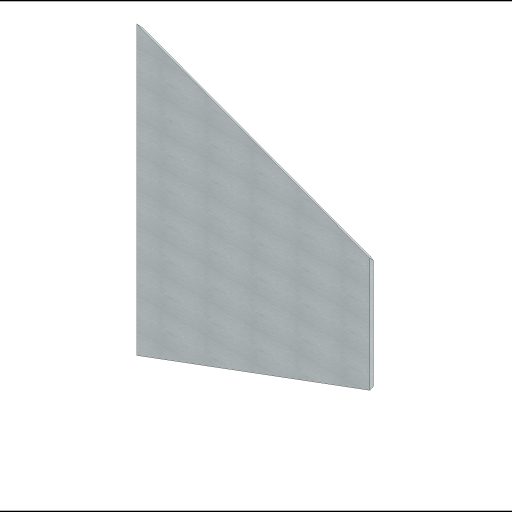
# Autodesk Inventor part: Wind Tunnel Inlet Body Single Panel
Saved by Autodesk Inventor 2023 (Build 270158000, 158)
## iProperties
Created: 2022-01-10
Part Number: Wind Tunnel Inlet Body Single Panel
Material: Wood (Oak)
Document SubType Name: Modeling
Designer: kamer
Density: 0.76 g/cm^3
Appearance: Wood - Painted White
Author: kamer
Autodesk Inventor part; units mm, degrees
ref_plane "YZ Plane" through (0, 0, 0) normal (1, 0, 0) x (0, 1, 0)
sketch "Sketch1" plane through (0, 0, 0) normal (0, 0, 1) x (1, 0, 0)
  line L0 (0, 0) -> (685.8, 0)
  line L1 (685.8, 0) -> (685.8, 838.2)
  line L2 (685.8, 838.2) -> (0, 838.2)
  line L3 (0, 838.2) -> (0, 0)
  line L4 (685.8, 254) -> (787.4, 254) construction
  line L5 (787.4, 254) -> (787.4, 584.2) construction
  line L6 (787.4, 584.2) -> (685.8, 584.2) construction
  line L7 (0, 838.2) -> (685.8, 584.2)
  line L8 (0, 0) -> (685.8, 254)
  dimension "d0" = 685.8
  dimension "d1" = 838.2
  dimension "d2" = 101.6
  dimension "d3" = 330.2
  dimension "d4" = 254
  constraints: 18 end point, 4 perpendicular, 2 parallel, 2 point on line, 1 horizontal
  measures "d0" distance of L2.end L1.end
  measures "d1" distance of L1.end L0.end
  measures "d2" distance of L4.start L4.end
  measures "d3" distance of L4.end L5.end
  measures "d4" distance between parallel lines of L0 L4
extrude "Extrusion1" add sketch "Sketch1" along normal blind 12.7 contours L3 L7 L1 L8
sketch "Sketch2" plane through (0, 0, 0) normal (-1, 0, 0) x (0, 0, 1)
  line L0 (12.7, 838.2) -> (12.7, 0) projected
  line L1 (12.7, 0) -> (0, 11.7954)
  line L2 (0, 838.2) -> (0, 0) projected
  line L3 (12.7, 0) -> (30.0327, 0) construction
  line L4 (12.7, 838.2) -> (0, 825.5)
  line L5 (12.7, 838.2) -> (30.6605, 838.2) construction
  line L6 (0, 838.2) -> (12.7, 838.2) projected
  line L7 (12.7, 838.2) -> (0, 838.2)
  line L8 (0, 838.2) -> (0, 825.5)
  line L9 (0, 0) -> (12.7, 0) projected
  line L10 (12.7, 0) -> (0, 0)
  line L11 (0, 0) -> (0, 11.7954)
  dimension "d7" = 137.115
  dimension "d8" = 135
  constraints: 16 end point, 3 horizontal, 2 equal length, 2 perpendicular, 2 point on line, 1 collinear
  measures "d7" angle of L3 L1
  measures "d8" angle of L4 L5
sketch "Sketch3" plane through (685.8, 254, 0) normal (1, 0, 0) x (0, 0, -1)
  line L0 (-12.7, -254) -> (-12.7, 0) projected
  line L1 (-12.7, 0) -> (0, 11.7954)
  line L2 (0, 0) -> (0, 330.2) projected
  line L3 (-12.7, 0) -> (4.6327, 0) construction
  line L4 (0, 11.7954) -> (0, 0)
  line L5 (0, 0) -> (-12.7, 0)
  line L6 (-12.7, 0) -> (-12.7, 330.2) projected
  line L7 (-12.7, 330.2) -> (0, 316.526)
  line L8 (0, 316.526) -> (0, 330.2)
  line L9 (0, 330.2) -> (-12.7, 330.2)
  point P0 (0, -254)
  dimension "d9" = 42.885
  constraints: 14 end point, 3 perpendicular, 3 point on line, 1 collinear, 1 equal length, 1 horizontal
  measures "d9" angle of L3 L1
loft "Loft1" cut profiles "Sketch3", "Sketch2" contours L1 L2 L5 / L9 L2 L1
sketch "Sketch4" plane through (685.8, 584.2, 12.7) normal (1, 0, 0) x (0, 0, -1)
  line L0 (0, 0) -> (0, 254) projected
  line L1 (0, 0) -> (12.7, -11.7954)
  line L2 (12.7, -318.4046) -> (12.7, 0) projected
  line L3 (0, 0) -> (17.3327, 0) construction
  line L4 (12.7, -11.7954) -> (12.7, 0)
  line L5 (12.7, 0) -> (0, 0)
  point P0 (12.7, -584.2)
  dimension "d14" = 42.885
  constraints: 8 end point, 1 collinear, 1 equal length, 1 horizontal, 1 perpendicular, 1 point on line
  measures "d14" angle of L1 L3
sketch "Sketch5" plane through (0, 11.7954, 0) normal (-1, 0, 0) x (0, 0, 1)
  line L0 (0, 826.4046) -> (12.7, 826.4046) projected
  line L1 (12.7, 826.4046) -> (0, 814.6093)
  line L2 (0, 572.4046) -> (0, 826.4046) projected
  line L3 (12.7, 826.4046) -> (30.0327, 826.4046) construction
  line L4 (0, 814.6093) -> (0, 826.4046)
  line L5 (0, 826.4046) -> (12.7, 826.4046)
  point P0 (0, -11.7954)
  dimension "d15" = 137.115
  constraints: 8 end point, 1 collinear, 1 equal length, 1 horizontal, 1 perpendicular, 1 point on line
  measures "d15" angle of L1 L3
loft "Loft2" cut profiles "Sketch5", "Sketch4"
ref_plane "Work Plane1" through (685.8, 0, 0) normal (0.923076, 0, -0.3846176) x (0, 1, 0)
ref_plane "Work Plane2" through (0, 419.1, 0) normal (0, 1, 0) x (-1, 0, 0)
sketch "Sketch7" plane through (0, 419.1, 0) normal (0, 1, 0) x (-1, 0, 0)
  line L0 (-685.8, 0) -> (0, 0) projected
  line L1 (-685.8, 0) -> (-680.7358, 12.7)
  line L2 (0, 12.7) -> (-685.8, 12.7) projected
  line L3 (-685.8, 0) -> (-672.1275, 0) construction
  line L4 (-680.7358, 12.7) -> (-685.8, 12.7)
  line L5 (-685.8, 12.7) -> (-685.8, 0)
  dimension "d26" = 68.26
  constraints: 8 end point, 1 collinear, 1 equal length, 1 horizontal, 1 perpendicular, 1 point on line
  measures "d26" angle of L3 L1
extrude "Extrusion3" cut sketch "Sketch7" against normal through all both and the other way through all
sketch "Sketch8" plane through (0, 419.1, 0) normal (0, 1, 0) x (-1, 0, 0)
  line L0 (-685.8, 0) -> (0, 0) projected
  line L1 (0, 0) -> (14.0129, 0) construction
  line L2 (0, 12.7) -> (-680.7358, 12.7) projected
  line L3 (0, 12.7) -> (-4.9988, 0)
  line L4 (0, 12.7) -> (13.6484, 12.7) construction
  line L5 (-4.9988, 0) -> (0, 0)
  line L6 (0, 12.7) -> (0, 0)
  dimension "d32" = 111.485
  constraints: 10 end point, 2 horizontal, 1 collinear, 1 equal length, 1 perpendicular, 1 point on line
  measures "d32" angle of L3 L4
extrude "Extrusion4" cut sketch "Sketch8" against normal through all both and the other way through all
sketch "Sketch10" plane through (680.7358, 252.1244, 12.7) normal (0.9288742, 0, 0.3703953) x (0.3703953, 0, -0.9288742)
  line L0 (13.6725, 13.671) -> (13.6725, 320.2803) projected
  line L1 (13.6725, 345.6803) -> (7.8432, 345.6803)
  line L2 (7.8432, 345.6803) -> (7.8432, -11.729)
  line L3 (7.8432, -11.729) -> (13.6725, -11.729)
  line L4 (13.6725, -11.729) -> (13.6725, 345.6803)
  point P0 (-240.3446, -252.1244)
  point P1 (13.6725, 13.671)
  point P2 (13.6725, 320.2803)
  dimension "d37" = 5.8293
  dimension "d38" = 25.4
  dimension "d39" = 25.4
  constraints: 8 end point, 2 parallel, 1 horizontal, 1 perpendicular, 1 point on line
  measures "d37" distance between parallel lines of L2 L0
  measures "d38" distance from line of L0.end L1
  measures "d39" distance from line of L3 L0.start
extrude "Extrusion6" cut sketch "Sketch10" against normal through all
body "Solid1"
